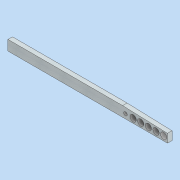
# Autodesk Inventor part: bodySidePlate
Saved by Autodesk Inventor 2021 (Build 250183000, 183)
## iProperties
Created: 2021-02-01
Part Number: bodySidePlate
Material: Generic
Document SubType Name: Modeling
Designer: garre
Density: 1 g/cm^3
Appearance: Default
Author: garre
Autodesk Inventor part; units mm, degrees
ref_plane "YZ Plane" through (0, 0, 0) normal (1, 0, 0) x (0, 1, 0)
ref_plane "XZ Plane" through (0, 0, 0) normal (0, 1, 0) x (-1, 0, 0)
ref_plane "XY Plane" through (0, 0, 0) normal (0, 0, 1) x (1, 0, 0)
sketch "Sketch1" plane through (0, 0, 0) normal (0, 0, 1) x (1, 0, 0)
  line L0 (0, 0) -> (647.7, 0)
  line L1 (647.7, 0) -> (647.7, 57.15)
  line L2 (647.7, 57.15) -> (0, 57.15)
  line L3 (0, 57.15) -> (0, 0)
  line L4 (647.7, 57.15) -> (901.7, 57.15)
  line L5 (901.7, 57.15) -> (901.7, 0)
  line L6 (901.7, 0) -> (647.7, 0)
  line L7 (647.7, 0) -> (647.7, 57.15)
  line L8 (647.7, 57.15) -> (901.7, 48.2801)
  dimension "d0" = 647.7
  dimension "d1" = 57.15
  dimension "d2" = 254
  dimension "d4" = 2
  constraints: 18 end point, 5 parallel, 2 horizontal, 2 perpendicular, 1 point on line
  measures "d0" distance of L1.end L2.end
  measures "d1" distance of L2.end L0.start
  measures "d2" distance of L1.end L4.end
  measures "d4" angle of L4 L8
extrude "Extrusion1" add sketch "Sketch1" along normal blind 25.4 contours L3 L2 L1 L0 | L1 L8 L5 L6
sketch "Sketch2" plane through (0, 0, 25.4) normal (0, 0, 1) x (1, 0, 0)
  line L0 (0, 0) -> (901.7, 0) projected
  line L1 (901.7, 0) -> (901.7, 25.4)
  line L2 (901.7, 25.4) -> (880.1227, 25.4)
  circle A0 centre (880.1227, 25.4) radius 17.399
  line L3 (880.1227, 25.4) -> (836.9681, 25.4)
  circle A1 centre (836.9681, 25.4) radius 17.399
  line L4 (836.9681, 25.4) -> (793.8135, 25.4)
  line L5 (793.8135, 25.4) -> (750.6589, 25.4)
  line L6 (750.6589, 25.4) -> (707.5043, 25.4)
  circle A2 centre (793.8135, 25.4) radius 17.399
  circle A3 centre (750.6589, 25.4) radius 17.399
  circle A4 centre (707.5043, 25.4) radius 17.399
  line L7 (901.7, 0) -> (901.7, 48.2801) projected
  line L8 (901.7, 0) -> (901.7, 48.2801)
  line L9 (707.5043, 25.4) -> (664.3497, 25.4)
  circle A5 centre (664.3497, 25.4) radius 9.525
  point P0 (787.6658, 25.1497)
  point P1 (813.0658, 25.1497)
  point P2 (838.4658, 25.1497)
  point P3 (863.8658, 25.1497)
  dimension "d7" = 25.4
  dimension "d8" = 21.5773
  dimension "d9" = 34.798
  dimension "d10" = 43.1546
  dimension "d13" = 19.05
  constraints: 16 end point, 6 centre point, 6 coincident, 5 collinear, 4 equal radius, 4 horizontal, 3 point on line
  measures "d7" distance of L0.end L1.end
  measures "d8" distance of L1.end L2.end
  measures "d9" diameter of A0
  measures "d10" distance of L3.start L3.end
  measures "d13" diameter of A5
extrude "Extrusion2" cut sketch "Sketch2" against normal up to surface (25.4 mm away)
equation "\"d0\" = bodyLengthUntilNut"
equation "\"d1\" = bodyHeight"
equation "\"d2\" = extensionLength"
equation "\"d4\" = postNutAngle"
equation "\"d5\" = woodThickness"
equation "\"d7\" = motorHolesOffset"
equation "\"d8\" = motorHoleEndOffset"
equation "\"d9\" = motorHoleDiameter"
equation "\"d10\" = motorHoleSeparation"
equation "\"d13\" = wireHoleDiameter"
equation "\"bodyLengthUntilNut\" = 647.7"
equation "\"postNutAngle\" = 2deg"
equation "\"woodThickness\" = 25.4"
equation "\"slantLength\" = 127"
equation "\"extensionLength\" = 254"
equation "\"bodyHeight\" = 57.15"
equation "\"motorHolesOffset\" = 25.4"
equation "\"motorHoleEndOffset\" = 21.5773"
equation "\"motorHoleDiameter\" = 34.798"
equation "\"motorHoleSeparation\" = 43.1546"
equation "\"wireHoleDiameter\" = 19.05"
body "Solid1"
